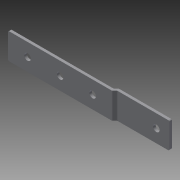
# Autodesk Inventor part: ConnectorHorizontal
Saved by Autodesk Inventor 2015 (Build 190159000, 159)
## iProperties
Created: 2015-04-22
Part Number: ConnectorHorizontal
Material: Generic
Document SubType Name: Modeling
Designer: krosie
Density: 1 g/cm^3
Appearance: Default
Author: krosie
Autodesk Inventor part; units mm, degrees
ref_plane "YZ Plane" through (0, 0, 0) normal (1, 0, 0) x (0, 1, 0)
ref_plane "XZ Plane" through (0, 0, 0) normal (0, 1, 0) x (-1, 0, 0)
ref_plane "XY Plane" through (0, 0, 0) normal (0, 0, 1) x (1, 0, 0)
sketch "Sketch1" plane through (0, 0, 0) normal (0, 0, 1) x (1, 0, 0)
  line L0 (0, 0) -> (80, 0)
  line L1 (80, 0) -> (82, 2)
  line L2 (82, 2) -> (122, 2)
  dimension "d0" = 80
  dimension "d1" = 135
  dimension "d2" = 40
  dimension "d3" = 2
  constraints: 6 end point, 1 horizontal, 1 parallel
  measures "d0" distance of L0.start L0.end
  measures "d1" angle of L1 L0
  measures "d2" distance of L1.end L2.end
  measures "d3" distance from line of L0 L1.end
sketch "Sketch3" plane through (0, 0, 0) normal (1, 0, 0) x (0, 1, 0)
  line L0 (0, 0) -> (0, -20)
  line L1 (0, -20) -> (2, -20)
  line L2 (2, -20) -> (2, 0)
  line L3 (2, 0) -> (0, 0)
  dimension "d13" = 20
  dimension "d14" = 2
  dimension "d15" = 20
  constraints: 8 end point, 2 vertical, 1 perpendicular
  measures "d13" distance of L0.start L0.end
  measures "d14" distance of L0.end L1.end
  measures "d15" distance of L1.end L2.end
sweep "Sweep1" add profiles "Sketch3" path "Sketch1"
fillet "Fillet3" radius 1 1 edges at (81.1716, 4, -10)
fillet "Fillet4" radius 1 1 edges at (82, 2, -10)
fillet "Fillet5" radius 1 1 edges at (80, 0, -10)
fillet "Fillet6" radius 1 1 edges at (79.1716, 2, -10)
hole "Hole1" at (15, 2, -10) direction (0, -1, 0) diameter 5 end through all
hole "Hole2" at (65, 2, -10) direction (0, -1, 0) diameter 5 end through all
hole "Hole3" at (112, 4, -10) direction (0, -1, 0) diameter 5 end through all
hole "Hole4" at (40, 2, -10) direction (0, -1, 0) diameter 5 end through all
fillet "Fillet7" radius 1 4 edges at (0, 1, 0) (0, 1, -20) (122, 3, 0) (122, 3, -20)
body "Solid1"
